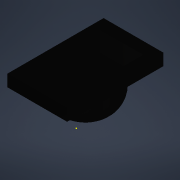
# Autodesk Inventor part: button
Saved by Autodesk Inventor 2022 (Build 260153000, 153)
## iProperties
Created: 2021-08-23
Part Number: button
Material: Gummi, Silikon
Document SubType Name: Modeling
Designer: Krillin
Density: 1.25 g/cm^3
Appearance: Eloxiert - Schwarz
Mass: 0.0489955 g
Surface Area: 0.959076 cm^2
Volume: 0.0462222 cm^3
Author: Krillin
Autodesk Inventor part; units mm, degrees
ref_plane "YZ Plane" through (0, 0, 0) normal (1, 0, 0) x (0, 1, 0)
ref_plane "XZ Plane" through (0, 0, 0) normal (0, 1, 0) x (-1, 0, 0)
ref_plane "XY Plane" through (0, 0, 0) normal (0, 0, 1) x (1, 0, 0)
sketch "Skizze1" plane through (0, 0, 0) normal (0, 1, 0) x (-1, 0, 0)
  circle A0 centre (2.7514, -3.3638) radius 2.05
  point P0 (0, 0)
  dimension "d0" = 4.1
  constraints: 1 centre point
  measures "d0" diameter of A0
extrude "Extrusion1" add sketch "Skizze1" along normal blind 2
fillet "Rundung1" radius 1.5 1 edges at (-0.7014, 0, -3.3638)
sketch "Skizze9" plane through (-2.7514, 2, -3.3638) normal (0, 1, 0) x (1, 0, 0)
  point P0 (2.7514, -3.3638)
sketch "Skizze10" plane through (-2.7514, 2, -3.3638) normal (0, 1, 0) x (1, 0, 0)
  line L0 (0, 0) -> (2.05, 0)
  line L1 (2.05, 0) -> (2.05, 3.3)
  line L2 (2.05, 3.3) -> (0, 3.3)
  line L3 (0, 3.3) -> (0, 0)
  line L4 (2.05, 3.3) -> (-2.05, 3.3)
  line L5 (-2.05, 3.3) -> (-2.05, -3.3)
  line L6 (-2.05, -3.3) -> (2.05, -3.3)
  line L7 (2.05, -3.3) -> (2.05, 3.3)
  point P0 (2.7514, -3.3638)
  point P1 (0, 3.3)
  dimension "d27" = 3.3
  dimension "d28" = 6.6
  constraints: 16 end point, 4 parallel, 2 horizontal, 2 perpendicular
  measures "d27" distance of L1.end L0.end
  measures "d28" distance of L5.end L4.end
extrude "Extrusion9" add sketch "Skizze10" along normal blind 0.8
sketch "Skizze12" plane through (-2.7514, 2.8, -3.3638) normal (0, 1, 0) x (1, 0, 0)
  line L0 (-0.0005, -0.0013) -> (-0.8005, -0.0013)
  line L1 (-0.8005, -0.0013) -> (-0.8005, 1.7987)
  line L2 (-0.8005, 1.7987) -> (-0.0005, 1.7987)
  line L3 (-0.0005, 1.7987) -> (-0.0005, -0.0013)
  line L4 (-0.8005, 1.7987) -> (0.7995, 1.7987)
  line L5 (0.7995, 1.7987) -> (0.7995, -1.8013)
  line L6 (0.7995, -1.8013) -> (-0.8005, -1.8013)
  line L7 (-0.8005, -1.8013) -> (-0.8005, 1.7987)
  point P0 (2.7514, -3.3638)
  dimension "d35" = 0.8
  dimension "d36" = 1.8
  dimension "d37" = 1.6
  dimension "d38" = 3.6
  constraints: 16 end point, 4 parallel, 2 horizontal, 2 perpendicular
  measures "d35" distance of L1.end L2.end
  measures "d36" distance of L0.end L1.end
  measures "d37" distance of L5.end L6.end
  measures "d38" distance of L4.end L5.end
extrude "Extrusion10" cut sketch "Skizze12" against normal blind 0.7
chamfer "Fase1" distance 0.7 angle 45 4 edges at (-1.9519, 2.8, -3.3625) (-3.5519, 2.8, -3.3625) (-2.7519, 2.8, -5.1625) (-2.7519, 2.8, -1.5625)
